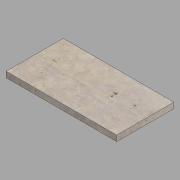
# Autodesk Inventor part: Stone base
Saved by Autodesk Inventor 2022.2 (Build 262287000, 287)
## iProperties
Created: 2021-12-06
Part Number: Stone base
Material: Limestone
Document SubType Name: Modeling
Designer: awelt
Density: 2.6 g/cm^3
Appearance: Kasota Gray
Mass: 8254.98 g
Surface Area: 2879.03 cm^2
Volume: 3174.99 cm^3
Author: awelt
Autodesk Inventor part; units mm, degrees
ref_plane "YZ Plane" through (0, 0, 0) normal (1, 0, 0) x (0, 1, 0)
ref_plane "XZ Plane" through (0, 0, 0) normal (0, 1, 0) x (-1, 0, 0)
ref_plane "XY Plane" through (0, 0, 0) normal (0, 0, 1) x (1, 0, 0)
sketch "Sketch1" plane through (0, 0, 0) normal (0, 1, 0) x (-1, 0, 0)
  line L0 (246.0625, -127) -> (-246.0625, -127)
  line L1 (-246.0625, -127) -> (-246.0625, 127)
  line L2 (-246.0625, 127) -> (246.0625, 127)
  line L3 (246.0625, 127) -> (246.0625, -127)
  line L4 (246.0625, -127) -> (-246.0625, 127) construction
  line L5 (-246.0625, -127) -> (246.0625, 127) construction
  point P0 (0, 0)
  dimension "d0" = 492.125
  dimension "d1" = 254
  constraints: 12 end point, 2 midpoint, 2 parallel, 1 horizontal, 1 perpendicular
  measures "d0" distance of L1.end L2.end
  measures "d1" distance of L0.end L1.end
extrude "Extrusion1" add sketch "Sketch1" along normal blind 25.4
body "Solid1"
